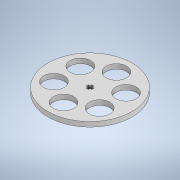
# Autodesk Inventor part: disc_mover
Saved by Autodesk Inventor 2020 (Build 240168000, 168)
## iProperties
Created: 2021-02-21
Part Number: disc_mover
Material: Generic
Document SubType Name: Modeling
Designer: HOME
Density: 1 g/cm^3
Appearance: Default
Author: HOME
Autodesk Inventor part; units mm, degrees
ref_plane "YZ Plane" through (0, 0, 0) normal (1, 0, 0) x (0, 1, 0)
ref_plane "XZ Plane" through (0, 0, 0) normal (0, 1, 0) x (-1, 0, 0)
ref_plane "XY Plane" through (0, 0, 0) normal (0, 0, 1) x (1, 0, 0)
sketch "Sketch1" plane through (0, 0, 0) normal (0, 1, 0) x (-1, 0, 0)
  circle A0 centre (0, 0) radius 35
  line L0 (0, 0) -> (0, -22)
  circle A1 centre (0, -22) radius 8.5
  circle A2 centre (-19.0526, -11) radius 8.5
  circle A3 centre (-19.0526, 11) radius 8.5
  circle A4 centre (0, 22) radius 8.5
  circle A5 centre (19.0526, 11) radius 8.5
  circle A6 centre (19.0526, -11) radius 8.5
  line L1 (-2.39, 0.895) -> (2.39, 0.895)
  line L2 (2.39, 0.895) -> (2.39, -0.895)
  line L3 (2.39, -0.895) -> (-2.39, -0.895)
  line L4 (-2.39, -0.895) -> (-2.39, 0.895)
  line L5 (-2.39, 0.895) -> (2.39, -0.895) construction
  line L6 (2.39, 0.895) -> (-2.39, -0.895) construction
  line L7 (-0.895, -2.39) -> (-0.895, 2.39)
  line L8 (0.895, -2.39) -> (-0.895, -2.39)
  line L9 (-0.895, 2.39) -> (0.895, 2.39)
  line L10 (0.895, 2.39) -> (0.895, -2.39)
  line L11 (-0.895, -2.39) -> (0.895, 2.39) construction
  line L12 (-0.895, 2.39) -> (0.895, -2.39) construction
  line L13 (2.39, -0.895) -> (-2.39, -0.895)
  line L14 (2.39, 0.895) -> (2.39, -0.895)
  line L15 (-2.39, -0.895) -> (-2.39, 0.895)
  line L16 (-2.39, 0.895) -> (2.39, 0.895)
  line L17 (2.39, -0.895) -> (-2.39, 0.895) construction
  line L18 (-2.39, -0.895) -> (2.39, 0.895) construction
  line L19 (0.895, 2.39) -> (0.895, -2.39)
  line L20 (-0.895, 2.39) -> (0.895, 2.39)
  line L21 (0.895, -2.39) -> (-0.895, -2.39)
  line L22 (-0.895, -2.39) -> (-0.895, 2.39)
  line L23 (0.895, 2.39) -> (-0.895, -2.39) construction
  line L24 (0.895, -2.39) -> (-0.895, 2.39) construction
  point P0 (-0.895, -0.895)
  point P1 (-0.895, 0.895)
  point P2 (0.895, 0.895)
  point P3 (0.895, -0.895)
  dimension "d0" = 70
  dimension "d1" = 22
  dimension "d2" = 17
  dimension "d5" = 360
  dimension "d9" = 4.78
  dimension "d10" = 1.79
  dimension "d13" = 360
  constraints: 50 end point, 12 coincident, 8 midpoint, 7 centre point, 2 parallel, 1 horizontal, 1 perpendicular, 1 vertical, 66 other
  measures "d0" diameter of A0
  measures "d1" distance of L0.start L0.end
  measures "d2" diameter of A1
  measures "d9" distance of L1.start L1.end
  measures "d10" distance of L1.end L2.end
extrude "Extrusion1" add sketch "Sketch1" along normal blind 4
body "Solid1"
